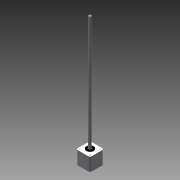
# Autodesk Inventor part: motor
Saved by Autodesk Inventor 2015 (Build 190159000, 159)
## iProperties
Created: 2015-01-29
Part Number: motor
Material: Generic
Document SubType Name: Modeling
Designer: Joseph
Density: 1 g/cm^3
Appearance: Default
Author: Joseph
Autodesk Inventor part; units mm, degrees
ref_plane "YZ Plane" through (0, 0, 0) normal (1, 0, 0) x (0, 1, 0)
ref_plane "XZ Plane" through (0, 0, 0) normal (0, 1, 0) x (-1, 0, 0)
ref_plane "XY Plane" through (0, 0, 0) normal (0, 0, 1) x (1, 0, 0)
sketch "Sketch1" plane through (0, 0, 0) normal (0, 0, 1) x (1, 0, 0)
  line L0 (17.5196, 21.1512) -> (-17.5142, 21.1512)
  line L1 (-21.1533, 17.5121) -> (-21.1533, -17.5122)
  line L2 (-17.5142, -21.1513) -> (17.5196, -21.1513)
  line L3 (21.1587, -17.5122) -> (21.1587, 17.5121)
  line L4 (21.1533, 21.1533) -> (-21.1467, -21.1467) construction
  line L5 (-21.1598, 21.1533) -> (21.1533, -21.1467) construction
  line L6 (-17.691, 21.078) -> (-21.08, 17.6889)
  line L7 (17.6964, 21.078) -> (21.0855, 17.6889)
  line L8 (21.0855, -17.689) -> (17.6964, -21.0781)
  line L9 (-17.691, -21.0781) -> (-21.08, -17.689)
  arc A0 (-17.5142, 21.1512) -> (-17.691, 21.078) centre (-17.5142, 20.9012) ccw
  arc A1 (-21.08, 17.6889) -> (-21.1533, 17.5121) centre (-20.9033, 17.5121) ccw
  arc A2 (17.6964, 21.078) -> (17.5196, 21.1512) centre (17.5196, 20.9012) ccw
  arc A3 (21.1587, 17.5121) -> (21.0855, 17.6889) centre (20.9087, 17.5121) ccw
  arc A4 (21.0855, -17.689) -> (21.1587, -17.5122) centre (20.9087, -17.5122) ccw
  arc A5 (17.5196, -21.1513) -> (17.6964, -21.0781) centre (17.5196, -20.9013) ccw
  arc A6 (-17.691, -21.0781) -> (-17.5142, -21.1513) centre (-17.5142, -20.9013) ccw
  arc A7 (-21.1533, -17.5122) -> (-21.08, -17.689) centre (-20.9033, -17.5122) ccw
  point P0 (0, 0)
  point P1 (-17.6177, 21.1512)
  point P2 (-21.1533, 17.6156)
  dimension "d0" = 42.3
  dimension "d1" = 42.3
  dimension "d2" = 5
  dimension "d3" = 45
  dimension "d4" = 0.25
  constraints: 20 end point, 16 point on circle, 16 tangent, 8 centre point, 7 equal radius, 6 point on line, 4 parallel, 3 equal length, 3 perpendicular, 1 horizontal
  measures "d0" distance of L5.end L4.end
  measures "d1" distance of L4.end L5.start
  measures "d2" distance of point (-17.618, 21.151) point (-21.153, 17.616)
  measures "d3" angle of L6 L0
  measures "d4" radius of A0
extrude "Extrusion1" add sketch "Sketch1" along normal blind 40
sketch "Sketch2" plane through (0, 0, 40) normal (0, 0, 1) x (1, 0, 0)
  circle A0 centre (0, 0) radius 11
  circle A1 centre (0, 0) radius 5
  dimension "d7" = 22
  dimension "d8" = 10
  constraints: 2 centre point, 2 coincident
  measures "d7" diameter of A0
  measures "d8" diameter of A1
extrude "Extrusion2" add sketch "Sketch2" along normal blind 2
sketch "Sketch3" plane through (0, 0, 40) normal (0, 0, 1) x (1, 0, 0)
  circle A0 centre (0, 0) radius 11 projected
  line L0 (-15.5, -15.5) -> (15.5, -15.5) construction
  line L1 (15.5, -15.5) -> (15.5, 15.5) construction
  line L2 (15.5, 15.5) -> (-15.5, 15.5) construction
  line L3 (-15.5, 15.5) -> (-15.5, -15.5) construction
  line L4 (-15.5, -15.5) -> (15.5, 15.5) construction
  line L5 (15.5, -15.5) -> (-15.5, 15.5) construction
  dimension "d11" = 31
  dimension "d12" = 31
  constraints: 12 end point, 4 coincident, 2 midpoint, 2 parallel, 1 horizontal, 1 perpendicular
  measures "d11" distance of L2.end L1.end
  measures "d12" distance of L1.end L0.end
hole "Hole1" at (-15.5, 15.5, 40) at (15.5, 15.5, 40) at (15.5, -15.5, 40) at (-15.5, -15.5, 40) direction (0, 0, -1) diameter 2.459 depth 4.5 tip angle 118 thread size "M3x0.5" class "6H" standard "ANSI Metric M Profile"
sketch "Sketch4" plane through (0, 0, 40) normal (0, 0, 1) x (1, 0, 0)
  circle A0 centre (0, 0) radius 5 projected
  circle A1 centre (0, 0) radius 4
  dimension "d20" = 8
  constraints: 1 centre point, 1 coincident
  measures "d20" diameter of A1
extrude "Extrusion3" add sketch "Sketch4" along normal blind 350 contours A1
body "Solid1"
